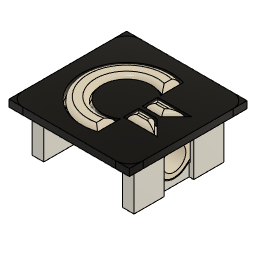
C-Logo_illuminated v12 (Autodesk Fusion 360 design; units mm, degrees)
Autodesk Fusion 360 part; units mm, degrees
sketch "Skizze1" plane through (0, 0, 0) normal (0, 0, 1) x (1, 0, 0)
  line L0 (10, 9.7) -> (-10, 9.7) construction
  line L1 (-10, 9.7) -> (-10, -9.7) construction
  line L2 (-10, -9.7) -> (10, -9.7) construction
  line L3 (10, -9.7) -> (10, 9.7) construction
  line L4 (10, 9.7) -> (-10, -9.7) construction
  line L5 (-10, 9.7) -> (10, -9.7) construction
  line L6 (10, 3.7) -> (2.72, 3.7)
  line L7 (6.68, 0.38) -> (2.72, 0.38)
  arc A0 (2.72, 9.2179) -> (2.72, -9.2179) centre (-0.3, 0) ccw
  arc A1 (2.72, 4.3554) -> (2.72, -4.3554) centre (-0.3, 0) ccw
  line L8 (10, 0) -> (-10, 0) construction
  line L9 (2.72, 9.2179) -> (2.72, 4.3554)
  line L10 (2.72, 3.7) -> (2.72, 0.38)
  line L11 (2.72, -4.3554) -> (2.72, -9.2179)
  line L12 (10, 3.7) -> (6.68, 0.38)
  line L13 (10, 3.7) -> (89.56, 3.7) construction
  line L14 (10, 3.7) -> (6.68, 0.38)
  line L15 (2.72, -0.38) -> (2.72, -3.7)
  line L16 (2.72, -3.7) -> (10, -3.7)
  line L17 (2.72, -0.38) -> (6.68, -0.38)
  line L18 (6.68, -0.38) -> (10, -3.7)
  line L19 (10, 12.7) -> (-10, 12.7)
  line L20 (-13, 9.7) -> (-13, -9.7)
  line L21 (-10, -12.7) -> (10, -12.7)
  line L22 (13, -9.7) -> (13, 9.7)
  line L23 (13, 12.7) -> (-13, -12.7) construction
  line L24 (-13, 12.7) -> (13, -12.7) construction
  arc A2 (-13, -9.7) -> (-10, -12.7) centre (-10, -9.7) ccw
  arc A3 (10, -12.7) -> (13, -9.7) centre (10, -9.7) ccw
  arc A4 (13, 9.7) -> (10, 12.7) centre (10, 9.7) ccw
  arc A5 (-10, 12.7) -> (-13, 9.7) centre (-10, 9.7) ccw
  line L25 (10, 3.7) -> (6.68, 0.38)
  line L26 (6.68, 0.38) -> (2.72, 0.38)
  line L27 (2.72, 3.7) -> (2.72, 0.38)
  line L28 (10, 3.7) -> (2.72, 3.7)
  line L29 (2.72, -3.7) -> (10, -3.7)
  line L30 (6.68, -0.38) -> (10, -3.7)
  line L31 (2.72, -0.38) -> (6.68, -0.38)
  line L32 (2.72, -0.38) -> (2.72, -3.7)
  arc A6 (2.72, 9.2179) -> (2.72, -9.2179) centre (-0.3, 0) ccw
  line L33 (2.72, -4.3554) -> (2.72, -9.2179)
  arc A7 (2.72, 4.3554) -> (2.72, -4.3554) centre (-0.3, 0) ccw
  line L34 (2.72, 9.2179) -> (2.72, 4.3554)
  dimension "d2" = 20
  dimension "d3" = 19.4
  dimension "d6" = 6
  dimension "d7" = 5.3
  dimension "d8" = 3.32
  dimension "d9" = 135
  dimension "d11" = 3
  dimension "d12" = 3
  dimension "d13" = 3
  dimension "d14" = 3
  dimension "d15" = 3
  dimension "d16" = 3
  dimension "d35" = 12.72
  constraint perpendicular L0 L1
  constraint parallel L0 L2
  constraint parallel L1 L3
  constraint horizontal L0
  constraint coincident L4 origin
  constraint coincident L5 origin
  constraint tangent L0 A0
  constraint tangent L1 A0
  constraint tangent L2 A0
  constraint perpendicular L2 L9
  constraint coincident L3 L6.start
  constraint coincident L6.end L9
  constraint perpendicular L6 L9
  constraint coincident L7.end L9
  constraint perpendicular L7 L9
  constraint coincident A0.end L9
  constraint coincident A1.end L9
  constraint concentric A0 A1
  constraint midpoint L3 L8.start
  constraint midpoint A0 L8.end
  constraint collinear L9 L10
  constraint collinear L10 L11
  constraint horizontal L13
  constraint coincident L12 L7.start
  constraint perpendicular L8 L15
  constraint coincident L3 L16.end
  constraint perpendicular L3 L16
  constraint perpendicular L15 L17
  constraint symmetric L7 L8 L17
  constraint symmetric L8 L10 L15
  constraint symmetric L6 L8 L16
  constraint symmetric L8 L12 L18
  constraint perpendicular L19 L20
  constraint parallel L19 L21
  constraint parallel L20 L22
  constraint horizontal L19
  constraint coincident L23 origin
  constraint coincident L24 origin
  constraint coincident L23.end L20
  constraint coincident L23.end L21
  constraint tangent L20 A2
  constraint tangent L21 A2
  constraint coincident L24.end L21
  constraint coincident L24.end L22
  constraint tangent L21 A3
  constraint tangent L22 A3
  constraint coincident L23.start L19
  constraint coincident L23.start L22
  constraint tangent L19 A4
  constraint tangent L22 A4
  constraint coincident L24.start L20
  constraint coincident L24.start L19
  constraint tangent L20 A5
  constraint tangent L19 A5
  measures "d2" distance of L1.end L2.end
  measures "d3" distance of L0.end L1.end
  measures "d6" distance of L0.start L6.start
  measures "d7" radius of A1
  measures "d8" distance of L6.end L7.end
  measures "d9" angle of L12 L13
  measures "d11" distance of L1 L20
  measures "d12" distance of L2 L21
  measures "d13" radius of A2
  measures "d14" radius of A3
  measures "d15" radius of A4
  measures "d16" radius of A5
  measures "d35" horizontal distance of L0.end A0.start
sketch "Skizze4" plane through (0, 0, 0) normal (0, 0, 1) x (1, 0, 0)
  arc A0 (2.72, 9.2179) -> (2.72, -9.2179) centre (-0.3, 0) ccw
  line L0 (2.72, 9.2179) -> (2.72, 4.3554)
  arc A1 (2.72, 4.3554) -> (2.72, -4.3554) centre (-0.3, 0) ccw
  line L1 (2.72, -4.3554) -> (2.72, -9.2179)
  line L2 (2.72, -3.7) -> (10, -3.7)
  line L3 (6.68, -0.38) -> (10, -3.7)
  line L4 (2.72, -0.38) -> (2.72, -3.7)
  line L5 (2.72, -0.38) -> (6.68, -0.38)
  line L6 (6.68, 0.38) -> (2.72, 0.38)
  line L7 (10, 3.7) -> (6.68, 0.38)
  line L8 (2.72, 3.7) -> (2.72, 0.38)
  line L9 (10, 3.7) -> (2.72, 3.7)
  line L10 (10, 9.7) -> (-10, 9.7)
  line L11 (10, -9.7) -> (10, 9.7)
  line L12 (-10, -9.7) -> (10, -9.7)
  line L13 (-10, 9.7) -> (-10, -9.7)
  line L14 (2.32, -5.0622) -> (2.32, -8.9233)
  arc A2 (2.32, 8.9233) -> (2.32, -8.9233) centre (-0.3, 0) ccw
  line L15 (2.32, 8.9233) -> (2.32, 5.0622)
  arc A3 (2.32, 5.0622) -> (2.32, -5.0622) centre (-0.3, 0) ccw
  line L16 (6.5143, 0.78) -> (3.12, 0.78)
  line L17 (3.12, 3.3) -> (3.12, 0.78)
  line L18 (9.0343, 3.3) -> (3.12, 3.3)
  line L19 (9.0343, 3.3) -> (6.5143, 0.78)
  line L20 (3.12, -3.3) -> (9.0343, -3.3)
  line L21 (6.5143, -0.78) -> (9.0343, -3.3)
  line L22 (3.12, -0.78) -> (6.5143, -0.78)
  line L23 (3.12, -0.78) -> (3.12, -3.3)
  dimension "d54" = 0.4
  dimension "d55" = -0.4
  dimension "d56" = -0.4
extrude "Extrusion7" add sketch "Skizze4" against normal blind 1 contours A0 L0 A1 L1 | L2 L3 L4 L5 | L6 L7 L8 L9 | A0 L0 A1 L1 L10 L11 L12 | A0 L10 L13 | A0 L12 L13 | L14 A2 L15 A3 | L16 L17 L18 L19 | L20 L21 L22 L23 makes body 1
extrude "Extrusion8" add sketch "Skizze4" along normal blind 2 contours L14 A2 L15 A3 | L16 L17 L18 L19 | L20 L21 L22 L23 bodies 1
fillet "Abrundung5" radius 1 1 edges at (-6, 0, 2) 3 faces at (-1.1284, 8.0389, 2) (6.2229, 2.46, 2) (6.2229, -2.46, 2) on bodies 1
sketch "Skizze5" plane through (10, 0, 0) normal (1, 0, 0) x (0, 1, 0)
  line L0 (9.7, 0) -> (-9.7, 0)
  line L1 (-9.7, 0) -> (-9.7, -1)
  line L2 (-9.7, -1) -> (9.7, -1)
  line L3 (9.7, -1) -> (9.7, 0)
  line L4 (9.7, -1) -> (-9.7, -1)
  line L5 (0, -1) -> (0, -9.1868) construction
  circle A0 centre (0, -4.5) radius 2.5
  line L6 (-9.7, -1) -> (-2.2348, -7.1936)
  line L7 (9.7, -1) -> (2.2348, -7.1936)
  arc A1 (-2.2348, -7.1936) -> (2.2348, -7.1936) centre (0, -4.5) ccw
  dimension "d62" = 5
  dimension "d63" = 3.5
  dimension "d64" = 7
  constraint midpoint L2 L5.start
  constraint perpendicular L0 L5
  constraint coincident L5 A0.centre
  constraint concentric A0 A1
  constraint coincident L1.end L2.start
  constraint tangent L6 A1
  constraint coincident L2.end L3.start
  constraint tangent L7 A1
  measures "d62" diameter of A0
  measures "d63" distance of L4 A0.centre
  measures "d64" diameter of A1
extrude "Extrusion9" add sketch "Skizze5" against normal blind 20 contours L2 L4 L6 L7 A1 bodies 1
extrude "Extrusion10" add sketch "Skizze1" along normal blind 1 separate body makes body 2
sketch "Skizze6" plane through (0, 0, 0) normal (0, 0, 1) x (-1, 0, 0)
  line L0 (-6.5143, 0.78) -> (-9.0343, 3.3)
  line L1 (-9.0343, 3.3) -> (-3.12, 3.3)
  line L2 (-3.12, 3.3) -> (-3.12, 0.78)
  line L3 (-3.12, 0.78) -> (-6.5143, 0.78)
  line L4 (-3.12, -3.3) -> (-9.0343, -3.3)
  line L5 (-9.0343, -3.3) -> (-6.5143, -0.78)
  line L6 (-6.5143, -0.78) -> (-3.12, -0.78)
  line L7 (-3.12, -0.78) -> (-3.12, -3.3)
  line L8 (-2.32, -8.9233) -> (-2.32, -5.0622)
  arc A0 (-2.32, -5.0622) -> (-2.32, 5.0622) centre (0.3, 0) ccw
  line L9 (-2.32, 5.0622) -> (-2.32, 8.9233)
  arc A1 (-2.32, -8.9233) -> (-2.32, 8.9233) centre (0.3, 0) ccw
  line L10 (10, -9.7) -> (10, 9.7)
  line L11 (10, 9.7) -> (-10, 9.7)
  line L12 (-10, 9.7) -> (-10, -9.7)
  line L13 (-10, -9.7) -> (10, -9.7)
  line L14 (10, 12.7) -> (-10, 12.7)
  arc A2 (-2.72, -4.3554) -> (-2.72, 4.3554) centre (0.3, 0) ccw
  line L15 (-2.72, 4.3554) -> (-2.72, 9.2179)
  arc A3 (-2.72, -9.2179) -> (-2.72, 9.2179) centre (0.3, 0) ccw
  line L16 (-2.72, -9.2179) -> (-2.72, -4.3554)
  line L17 (-10, -3.7) -> (-2.72, -3.7)
  line L18 (-10, -3.7) -> (-6.68, -0.38)
  line L19 (-6.68, -0.38) -> (-2.72, -0.38)
  line L20 (-2.72, -3.7) -> (-2.72, -0.38)
  line L21 (-2.72, 0.38) -> (-6.68, 0.38)
  line L22 (-6.68, 0.38) -> (-10, 3.7)
  line L23 (-2.72, 3.7) -> (-10, 3.7)
  line L24 (-2.72, 0.38) -> (-2.72, 3.7)
  line L25 (-13, 9.7) -> (-13, -9.7)
  line L26 (-10, -12.7) -> (10, -12.7)
  line L27 (13, -9.7) -> (13, 9.7)
  line L28 (13, -9.7) -> (13, -12.7)
  line L29 (13, -12.7) -> (10, -12.7)
  line L30 (-10, -12.7) -> (-13, -12.7)
  line L31 (-13, -12.7) -> (-13, -9.7)
  line L32 (-13, 9.7) -> (-13, 12.7)
  line L33 (-13, 12.7) -> (-10, 12.7)
  line L34 (10, 12.7) -> (13, 12.7)
  line L35 (13, 12.7) -> (13, 9.7)
  constraint coincident L27.start L28.start
  constraint perpendicular L26 L28
  constraint coincident L26.end L29.end
  constraint perpendicular L28 L29
  constraint coincident L26.start L30.start
  constraint perpendicular L25 L30
  constraint coincident L25.end L31.end
  constraint perpendicular L30 L31
  constraint coincident L25.start L32.start
  constraint perpendicular L14 L32
  constraint coincident L14.end L33.end
  constraint perpendicular L32 L33
  constraint coincident L14.start L34.start
  constraint perpendicular L27 L34
  constraint coincident L27.end L35.end
  constraint perpendicular L34 L35
extrude "Extrusion11" add sketch "Skizze6" along normal blind 1.5 separate body contours L10 L13 A3 | L10 L11 A3 | L11 L12 L13 A2 L15 A3 L16 | L14 L25 L26 L27 L28 L29 L30 L31 L32 L33 L34 L35 makes body 3
extrude "Extrusion12" add 1 faces at (7.5733, -8.5393, 1) along direction (0, 0, 1) blind 0.5 on bodies 2 bodies 2
sketch "Skizze7" plane through (10, 0, 0) normal (1, 0, 0) x (0, 1, 0)
  circle A0 centre (0, -4.5) radius 2.5
  line L0 (9.7, 0) -> (-9.7, 0)
  line L1 (-9.7, 0) -> (-9.7, -1)
  line L2 (-9.7, -1) -> (-2.2348, -7.1936)
  arc A1 (-2.2348, -7.1936) -> (2.2348, -7.1936) centre (0, -4.5) ccw
  line L3 (2.2348, -7.1936) -> (9.7, -1)
  line L4 (9.7, -1) -> (9.7, 0)
  arc A2 (-2.2348, -7.1936) -> (2.2348, -7.1936) centre (0, -4.5) ccw
  line L5 (-9.7, -1) -> (-2.2348, -7.1936)
  line L6 (9.7, -1) -> (2.2348, -7.1936)
  line L7 (-9.7, -1) -> (-2.2348, -7.1936)
  arc A3 (-2.2348, -7.1936) -> (2.2348, -7.1936) centre (0, -4.5) ccw
  line L8 (9.7, -1) -> (2.2348, -7.1936)
  line L9 (3.1926, -8.348) -> (9.7, -2.949)
  line L10 (-9.7, -2.949) -> (-3.1926, -8.348)
  arc A4 (-3.1926, -8.348) -> (3.1926, -8.348) centre (0, -4.5) ccw
  line L11 (-9.7, -1.2599) -> (-2.3625, -7.3475)
  arc A5 (-2.3625, -7.3475) -> (2.3625, -7.3475) centre (0, -4.5) ccw
  line L12 (2.3625, -7.3475) -> (9.7, -1.2599)
  line L13 (-9.7, -1.2599) -> (-9.7, -2.949)
  line L14 (9.7, -1.2599) -> (9.7, -2.949)
  line L15 (-9.7, -2.949) -> (-9.7, -9.5)
  line L16 (-9.7, -9.5) -> (0, -9.5)
  line L17 (0, -9.5) -> (9.7, -9.5)
  line L18 (9.7, -9.5) -> (9.7, -2.949)
  line L19 (-9.7, -1.2599) -> (-3.2, -1.2599)
  line L20 (-3.2, -1.2599) -> (-3.2, -9.5)
  line L21 (-3.2, -9.5) -> (-9.7, -9.5)
  line L22 (-9.7, -9.5) -> (-9.7, -1.2599)
  line L23 (9.7, -1.2599) -> (3.2, -1.2599)
  line L24 (3.2, -1.2599) -> (3.2, -9.5)
  line L25 (3.2, -9.5) -> (9.7, -9.5)
  line L26 (9.7, -9.5) -> (9.7, -1.2599)
  dimension "d75" = 0.2
  dimension "d76" = 1.3
  dimension "d77" = 9.7
  dimension "d78" = 19.4
  dimension "d86" = 6.5
  dimension "d87" = 6.5
  constraint parallel L3 L9
  constraint parallel L2 L10
  constraint concentric A1 A4
  constraint tangent L9 A4
  constraint tangent L10 A4
  constraint parallel L2 L11
  constraint concentric A1 A5
  constraint parallel L3 L12
  constraint tangent L11 A5
  constraint tangent A5 L12
  constraint vertical L13
  constraint parallel L13 L14
  constraint parallel L13 L15
  constraint midpoint A4 L16.end
  constraint tangent A4 L16
  constraint tangent A4 L17
  constraint perpendicular L14 L17
  constraint perpendicular L17 L18
  constraint horizontal L19
  constraint vertical L20
  constraint horizontal L21
  constraint vertical L22
  constraint coincident L16 L20.end
  constraint horizontal L23
  constraint vertical L24
  constraint horizontal L25
  constraint vertical L26
  constraint coincident L17 L24.end
  measures "d75" distance of L3 L12
  measures "d76" distance of L10 L11
  measures "d77" horizontal distance of L11.start origin
  measures "d78" distance of L15.end L17.end
  measures "d86" distance of L15 L20
  measures "d87" distance of L18 L24
extrude "Extrusion13" add sketch "Skizze7" against normal blind 20 separate body contours L9 L12 L14 L24 L26 | L10 L11 L13 L20 L22 | L9 L10 A4 L11 A5 L12 L20 L24 makes body 4
extrude "Extrusion14" add sketch "Skizze7" against normal blind 1.5 contours L9 L17 L18 L24 L25 L26 | L10 L15 L16 L20 L21 L22 | L9 A4 L17 L24 | L10 A4 L16 L20 bodies 4
extrude "Extrusion15" add sketch "Skizze7" against normal blind 1.5 from surface at -18.5 contours L9 L17 L18 L24 L25 L26 | L10 L15 L16 L20 L21 L22 | L9 A4 L17 L24 | L10 A4 L16 L20 bodies 4
extrude "Extrusion16" add sketch "Skizze7" along normal blind 1 contours L3 L6 L8 L12 L23 L24 | L3 L6 L8 L23 L24 | L2 L5 L7 L19 L20 | L2 L5 L7 L11 L19 L20 | L9 L12 L14 L24 L26 | L10 L11 L13 L20 L22 | L9 L17 L18 L24 L25 L26 | L10 L15 L16 L20 L21 L22 bodies 4
extrude "Extrusion17" add sketch "Skizze7" against normal blind 1 from surface at -20 contours L3 L6 L8 L12 L23 L24 | L3 L6 L8 L23 L24 | L2 L5 L7 L19 L20 | L2 L5 L7 L11 L19 L20 | L9 L12 L14 L24 L26 | L10 L11 L13 L20 L22 | L9 L17 L18 L24 L25 L26 | L10 L15 L16 L20 L21 L22 bodies 4
move_face "Flächen versetzen1" offset -0.25 2 faces at (-10, 5.3667, -3.0575) (-10, -5.3667, -3.0575) on bodies 4
move_face "Flächen versetzen2" offset -0.25 2 faces at (10, -5.3667, -3.0575) (10, 5.3667, -3.0575) on bodies 4
equation "baselineA = 20 mm"
equation "d2 = baselineA"
equation "d3 = baselineA * 0.97"
equation "d6 = baselineA * 0.3"
equation "d7 = baselineA * 0.53 / 2"
equation "d8 = baselineA * 0.166"
equation "framedistance = 3 mm"
equation "d11 = framedistance"
equation "d12 = framedistance"
equation "d13 = framedistance"
equation "d14 = framedistance"
equation "d15 = framedistance"
equation "d16 = framedistance"
equation "height_logo = 5 mm"
equation "height_baseplate = 5 mm"
equation "height_below = 2 mm"
equation "distance_baseplate = 0.0 mm"
equation "d26 = -distance_baseplate"
equation "d27 = -distance_baseplate"
equation "d34 = -distance_baseplate"
equation "d35 = baselineA * 0.636"
equation "d65 = -baselineA"
named bodies: "illuminated body", "face plate rounded", "face plate 1.5", "reflector"
